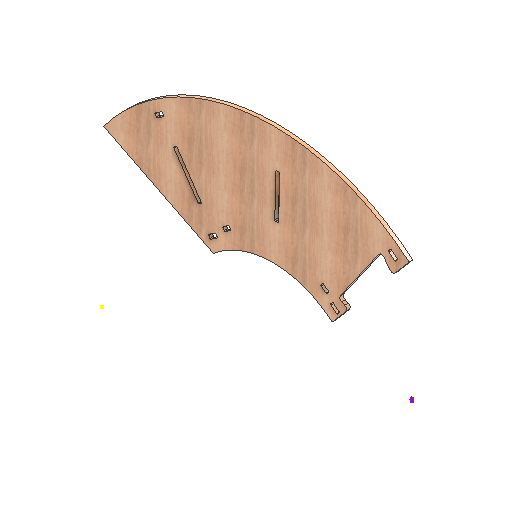
# Autodesk Inventor part: Platform B4
Saved by Autodesk Inventor 2021 (Build 250183000, 183)
## iProperties
Created: 2020-05-09
Part Number: Platform B4
Material: Wood (Birch)
Document SubType Name: Modeling
Designer: Dan Wikman
Density: 0.55 g/cm^3
Appearance: Birch - Natural Polished
Mass: 6310.79 g
Surface Area: 13696.6 cm^2
Volume: 11474.2 cm^3
Autodesk Inventor part; units mm, degrees
(part 1 of 2)
ref_plane "YZ Plane" through (0, 0, 0) normal (1, 0, 0) x (0, 1, 0)
ref_plane "XZ Plane" through (0, 0, 0) normal (0, 1, 0) x (-1, 0, 0)
ref_plane "XY Plane" through (0, 0, 0) normal (0, 0, 1) x (1, 0, 0)
sketch "Sketch1" plane through (0, 0, 0) normal (0, 0, 1) x (1, 0, 0)
  point P0 (0, 0)
sketch "CONTOURS" plane through (0, 0, 0) normal (0, 0, 1) x (1, 0, 0)
  line L0 (890.613, 255.6505) -> (890.613, 225.6505)
  line L1 (1985, 997.9541) -> (1985, 982.2281)
  arc A0 (1985, 982.2281) -> (1987, 980.2277) centre (1987, 982.2277) ccw
  line L2 (1987, 980.2277) -> (2103, 980.2277)
  arc A1 (2103, 980.2277) -> (2105, 982.2277) centre (2103, 982.2277) ccw
  line L3 (2105, 982.2277) -> (2105, 988.2874)
  arc A2 (2105, 988.2874) -> (2103.1661, 990.2805) centre (2103, 988.2874) ccw
  line L4 (2103.1661, 990.2805) -> (1987.1661, 999.9472)
  arc A3 (1987.1661, 999.9472) -> (1985, 997.9541) centre (1987, 997.9541) ccw
  line L5 (2105.3322, 1032.9996) -> (2105.3322, 1017.2736)
  arc A4 (2103.1661, 1015.2805) -> (2105.3322, 1017.2736) centre (2103.3322, 1017.2736) ccw
  line L6 (2103.1661, 1015.2805) -> (1987.1661, 1024.9472)
  arc A5 (1985.3322, 1026.9403) -> (1987.1661, 1024.9472) centre (1987.3322, 1026.9403) ccw
  line L7 (1985.3322, 1026.9403) -> (1985.3322, 1033)
  arc A6 (1987.3322, 1035) -> (1985.3322, 1033) centre (1987.3322, 1033) ccw
  line L8 (1987.3322, 1035) -> (2103.3322, 1035)
  arc A7 (2105.3322, 1032.9996) -> (2103.3322, 1035) centre (2103.3322, 1033) ccw
  line L9 (2125, 982.2281) -> (2125, 997.9541)
  arc A8 (2127.1661, 999.9472) -> (2125, 997.9541) centre (2127, 997.9541) ccw
  line L10 (2127.1661, 999.9472) -> (2243.1661, 990.2805)
  arc A9 (2245, 988.2874) -> (2243.1661, 990.2805) centre (2243, 988.2874) ccw
  line L11 (2245, 988.2874) -> (2245, 982.2277)
  arc A10 (2243, 980.2277) -> (2245, 982.2277) centre (2243, 982.2277) ccw
  line L12 (2243, 980.2277) -> (2127, 980.2277)
  arc A11 (2125, 982.2281) -> (2127, 980.2277) centre (2127, 982.2277) ccw
  line L13 (2265, 902.2281) -> (2265, 917.9541)
  arc A12 (2267.1661, 919.9472) -> (2265, 917.9541) centre (2267, 917.9541) ccw
  line L14 (2267.1661, 919.9472) -> (2383.1661, 910.2805)
  line L15 (2385, 908.2874) -> (2385, 902.2277)
  arc A13 (2383, 900.2277) -> (2385, 902.2277) centre (2383, 902.2277) ccw
  line L16 (2383, 900.2277) -> (2267, 900.2277)
  arc A14 (2265, 902.2281) -> (2267, 900.2277) centre (2267, 902.2277) ccw
  line L17 (2385.3322, 952.9996) -> (2385.3322, 937.2736)
  arc A15 (2383.1661, 935.2805) -> (2385.3322, 937.2736) centre (2383.3322, 937.2736) ccw
  line L18 (2383.1661, 935.2805) -> (2267.1661, 944.9472)
  arc A16 (2265.3322, 946.9403) -> (2267.1661, 944.9472) centre (2267.3322, 946.9403) ccw
  line L19 (2265.3322, 946.9403) -> (2265.3322, 953)
  arc A17 (2267.3322, 955) -> (2265.3322, 953) centre (2267.3322, 953) ccw
  line L20 (2267.3322, 955) -> (2383.3322, 955)
  arc A18 (2385.3322, 952.9996) -> (2383.3322, 955) centre (2383.3322, 953) ccw
  line L21 (2265, 1077.9541) -> (2265, 1062.2281)
  arc A19 (2265, 1062.2281) -> (2267, 1060.2277) centre (2267, 1062.2277) ccw
  line L22 (2267, 1060.2277) -> (2383, 1060.2277)
  arc A20 (2383, 1060.2277) -> (2385, 1062.2277) centre (2383, 1062.2277) ccw
  line L23 (2385, 1062.2277) -> (2385, 1068.2874)
  arc A21 (2385, 1068.2874) -> (2383.1661, 1070.2805) centre (2383, 1068.2874) ccw
  line L24 (2383.1661, 1070.2805) -> (2267.1661, 1079.9472)
  arc A22 (2267.1661, 1079.9472) -> (2265, 1077.9541) centre (2267, 1077.9541) ccw
  line L25 (2385.3322, 1112.9996) -> (2385.3322, 1097.2736)
  arc A23 (2383.1661, 1095.2805) -> (2385.3322, 1097.2736) centre (2383.3322, 1097.2736) ccw
  line L26 (2383.1661, 1095.2805) -> (2267.1661, 1104.9472)
  arc A24 (2265.3322, 1106.9403) -> (2267.1661, 1104.9472) centre (2267.3322, 1106.9403) ccw
  line L27 (2265.3322, 1106.9403) -> (2265.3322, 1113)
  arc A25 (2267.3322, 1115) -> (2265.3322, 1113) centre (2267.3322, 1113) ccw
  line L28 (2267.3322, 1115) -> (2383.3322, 1115)
  arc A26 (2385.3322, 1112.9996) -> (2383.3322, 1115) centre (2383.3322, 1113) ccw
  line L29 (2245.3322, 1112.9996) -> (2245.3322, 1097.2736)
  arc A27 (2243.1661, 1095.2805) -> (2245.3322, 1097.2736) centre (2243.3322, 1097.2736) ccw
  line L30 (2243.1661, 1095.2805) -> (2127.1661, 1104.9472)
  arc A28 (2125.3322, 1106.9403) -> (2127.1661, 1104.9472) centre (2127.3322, 1106.9403) ccw
  line L31 (2125.3322, 1106.9403) -> (2125.3322, 1113)
  arc A29 (2127.3322, 1115) -> (2125.3322, 1113) centre (2127.3322, 1113) ccw
  line L32 (2127.3322, 1115) -> (2243.3322, 1115)
  arc A30 (2245.3322, 1112.9996) -> (2243.3322, 1115) centre (2243.3322, 1113) ccw
  line L33 (2125, 1062.2281) -> (2125, 1077.9541)
  arc A31 (2127.1661, 1079.9472) -> (2125, 1077.9541) centre (2127, 1077.9541) ccw
  line L34 (2127.1661, 1079.9472) -> (2243.1661, 1070.2805)
  arc A32 (2245, 1068.2874) -> (2243.1661, 1070.2805) centre (2243, 1068.2874) ccw
  line L35 (2245, 1068.2874) -> (2245, 1062.2277)
  arc A33 (2243, 1060.2277) -> (2245, 1062.2277) centre (2243, 1062.2277) ccw
  line L36 (1397.2136, 921.0635) -> (1428.3528, 880.2176)
  arc A34 (1428.3528, 880.2176) -> (1450.9296, 879.6147) centre (1439.884, 889.0085) ccw
  line L37 (1450.9296, 879.6147) -> (1520.8494, 961.8291)
  arc A35 (1520.8494, 961.8291) -> (24.3664, 789.4308) centre (853.2136, 175.9412) ccw
  line L38 (24.3664, 789.4308) -> (562.1144, 519.2117)
  arc A36 (1144.4223, 519.2117) -> (562.1144, 519.2117) centre (853.2684, 176.0899) ccw
  line L39 (1144.4223, 519.2117) -> (1211.5255, 598.1141)
  arc A37 (1211.5255, 598.1141) -> (1206.0707, 620.8867) centre (1200.4798, 607.5079) ccw
  line L40 (1206.0707, 620.8867) -> (1190.5072, 627.3906)
  arc A38 (1183.7728, 650.5625) -> (1190.5072, 627.3906) centre (1196.4836, 641.6921) ccw
  line L41 (1183.7728, 650.5625) -> (1372.1762, 920.5366)
  arc A39 (1397.2136, 921.0635) -> (1372.1762, 920.5366) centre (1384.8871, 911.6663) ccw
  line L42 (2243, 1060.2277) -> (2127, 1060.2277)
  arc A40 (2125, 1062.2281) -> (2127, 1060.2277) centre (2127, 1062.2277) ccw
  line L43 (1985, 1077.9541) -> (1985, 1062.2281)
  arc A41 (1985, 1062.2281) -> (1987, 1060.2277) centre (1987, 1062.2277) ccw
  line L44 (1987, 1060.2277) -> (2103, 1060.2277)
  arc A42 (2103, 1060.2277) -> (2105, 1062.2277) centre (2103, 1062.2277) ccw
  line L45 (2105, 1062.2277) -> (2105, 1068.2874)
  arc A43 (2105, 1068.2874) -> (2103.1661, 1070.2805) centre (2103, 1068.2874) ccw
  line L46 (2103.1661, 1070.2805) -> (1987.1661, 1079.9472)
  arc A44 (1987.1661, 1079.9472) -> (1985, 1077.9541) centre (1987, 1077.9541) ccw
  line L47 (2385.3322, 1032.9996) -> (2385.3322, 1017.2736)
  arc A45 (2383.1661, 1015.2805) -> (2385.3322, 1017.2736) centre (2383.3322, 1017.2736) ccw
  line L48 (2383.1661, 1015.2805) -> (2267.1661, 1024.9472)
  arc A46 (2265.3322, 1026.9403) -> (2267.1661, 1024.9472) centre (2267.3322, 1026.9403) ccw
  line L49 (2265.3322, 1026.9403) -> (2265.3322, 1033)
  arc A47 (2267.3322, 1035) -> (2265.3322, 1033) centre (2267.3322, 1033) ccw
  line L50 (2267.3322, 1035) -> (2383.3322, 1035)
  arc A48 (2385.3322, 1032.9996) -> (2383.3322, 1035) centre (2383.3322, 1033) ccw
  line L51 (2245.3322, 1032.9996) -> (2245.3322, 1017.2736)
  arc A49 (2243.1661, 1015.2805) -> (2245.3322, 1017.2736) centre (2243.3322, 1017.2736) ccw
  line L52 (2243.1661, 1015.2805) -> (2127.1661, 1024.9472)
  arc A50 (1985.3322, 866.9403) -> (1987.1661, 864.9472) centre (1987.3322, 866.9403) ccw
  arc A51 (2125.3322, 1026.9403) -> (2127.1661, 1024.9472) centre (2127.3322, 1026.9403) ccw
  line L53 (2125.3322, 1026.9403) -> (2125.3322, 1033)
  line L54 (2153.8888, 619.2359) -> (2163.4719, 633.117)
  arc A52 (2185.9832, 634.7957) -> (2163.4719, 633.117) centre (2175.4045, 624.8791) ccw
  line L55 (2185.9832, 634.7957) -> (2411.1355, 394.6117)
  arc A53 (2406.7717, 371.5944) -> (2411.1355, 394.6117) centre (2400.5567, 384.695) ccw
  line L56 (2406.7717, 371.5944) -> (2360.367, 349.5799)
  arc A54 (2360.367, 349.5799) -> (2354.7432, 326.1016) centre (2367.0105, 335.5759) ccw
  line L57 (2354.7432, 326.1016) -> (2420.766, 240.6152)
  arc A55 (991.9076, 405.3519) -> (2420.766, 240.6152) centre (1790.9625, 1056.9921) ccw
  line L58 (991.9076, 405.3519) -> (1516.221, 700.5434)
  arc A56 (1516.221, 700.5434) -> (2065.5544, 700.5434) centre (1790.8877, 1057.1243) ccw
  line L59 (2065.5544, 700.5434) -> (2128.8659, 618.5677)
  arc A57 (2128.8659, 618.5677) -> (2153.8888, 619.2359) centre (2141.1332, 628.042) ccw
  arc A58 (2127.3322, 1035) -> (2125.3322, 1033) centre (2127.3322, 1033) ccw
  line L60 (2127.3322, 1035) -> (2243.3322, 1035)
  arc A59 (2245.3322, 1032.9996) -> (2243.3322, 1035) centre (2243.3322, 1033) ccw
  line L61 (2105.3322, 1112.9996) -> (2105.3322, 1097.2736)
  arc A60 (2103.1661, 1095.2805) -> (2105.3322, 1097.2736) centre (2103.3322, 1097.2736) ccw
  line L62 (2103.1661, 1095.2805) -> (1987.1661, 1104.9472)
  arc A61 (1985.3322, 1106.9403) -> (1987.1661, 1104.9472) centre (1987.3322, 1106.9403) ccw
  line L63 (1985.3322, 1106.9403) -> (1985.3322, 1113)
  arc A62 (1987.3322, 1115) -> (1985.3322, 1113) centre (1987.3322, 1113) ccw
  line L64 (1987.3322, 1115) -> (2103.3322, 1115)
  arc A63 (2105.3322, 1112.9996) -> (2103.3322, 1115) centre (2103.3322, 1113) ccw
  line L65 (2245.3322, 952.9996) -> (2245.3322, 937.2736)
  arc A64 (2243.1661, 935.2805) -> (2245.3322, 937.2736) centre (2243.3322, 937.2736) ccw
  line L66 (2243.1661, 935.2805) -> (2127.1661, 944.9472)
  arc A65 (2125.3322, 946.9403) -> (2127.1661, 944.9472) centre (2127.3322, 946.9403) ccw
  line L67 (2125.3322, 946.9403) -> (2125.3322, 953)
  arc A66 (2127.3322, 955) -> (2125.3322, 953) centre (2127.3322, 953) ccw
  line L68 (2127.3322, 955) -> (2243.3322, 955)
  arc A67 (2245.3322, 952.9996) -> (2243.3322, 955) centre (2243.3322, 953) ccw
  arc A68 (2385, 908.2874) -> (2383.1661, 910.2805) centre (2383, 908.2874) ccw
  arc A69 (113.8436, 518.7397) -> (113.8436, 526.7397) centre (113.8436, 522.7397) ccw
  line L69 (113.8436, 526.7397) -> (113.8436, 528.7397)
  line L70 (113.8436, 528.7397) -> (472.3436, 528.7397)
  line L71 (472.3436, 528.7397) -> (472.3436, 526.7397)
  arc A70 (472.3436, 526.7397) -> (472.3436, 518.7397) centre (472.3436, 522.7397) ccw
  line L72 (472.3436, 518.7397) -> (490.3436, 518.7397)
  line L73 (490.3436, 518.7397) -> (490.3436, 488.7397)
  line L74 (490.3436, 488.7397) -> (472.3436, 488.7397)
  arc A71 (472.3436, 488.7397) -> (472.3436, 480.7397) centre (472.3436, 484.7397) ccw
  line L75 (472.3436, 480.7397) -> (472.3436, 428.7397)
  line L76 (472.3436, 428.7397) -> (301.0936, 428.7397)
  arc A72 (301.0936, 428.7397) -> (293.0936, 428.7397) centre (297.0936, 428.7397) ccw
  line L77 (293.0936, 428.7397) -> (293.0936, 410.7397)
  line L78 (293.0936, 410.7397) -> (263.0936, 410.7397)
  line L79 (263.0936, 410.7397) -> (263.0936, 428.7397)
  arc A73 (263.0936, 428.7397) -> (255.0936, 428.7397) centre (259.0936, 428.7397) ccw
  line L80 (255.0936, 428.7397) -> (113.8436, 428.7397)
  line L81 (113.8436, 428.7397) -> (113.8436, 480.7397)
  arc A74 (113.8436, 480.7397) -> (113.8436, 488.7397) centre (113.8436, 484.7397) ccw
  line L82 (113.8436, 488.7397) -> (95.8436, 488.7397)
  line L83 (95.8436, 488.7397) -> (95.8436, 518.7397)
  line L84 (95.8436, 518.7397) -> (113.8436, 518.7397)
  arc A75 (87.6316, 255.6505) -> (87.6316, 263.6505) centre (87.6316, 259.6505) ccw
  line L85 (87.6316, 263.6505) -> (87.6316, 265.6505)
  line L86 (87.6316, 265.6505) -> (446.1316, 265.6505)
  line L87 (446.1316, 265.6505) -> (446.1316, 263.6505)
  arc A76 (446.1316, 263.6505) -> (446.1316, 255.6505) centre (446.1316, 259.6505) ccw
  line L88 (446.1316, 255.6505) -> (464.1316, 255.6505)
  line L89 (464.1316, 255.6505) -> (464.1316, 225.6505)
  line L90 (464.1316, 225.6505) -> (446.1316, 225.6505)
  arc A77 (446.1316, 225.6505) -> (446.1316, 217.6505) centre (446.1316, 221.6505) ccw
  line L91 (446.1316, 217.6505) -> (446.1316, 165.6505)
  line L92 (446.1316, 165.6505) -> (274.8816, 165.6505)
  arc A78 (274.8816, 165.6505) -> (266.8816, 165.6505) centre (270.8816, 165.6505) ccw
  line L93 (266.8816, 165.6505) -> (266.8816, 147.6505)
  line L94 (266.8816, 147.6505) -> (236.8816, 147.6505)
  line L95 (236.8816, 147.6505) -> (236.8816, 165.6505)
  arc A79 (236.8816, 165.6505) -> (228.8816, 165.6505) centre (232.8816, 165.6505) ccw
  line L96 (228.8816, 165.6505) -> (87.6316, 165.6505)
  line L97 (87.6316, 165.6505) -> (87.6316, 217.6505)
  arc A80 (87.6316, 217.6505) -> (87.6316, 225.6505) centre (87.6316, 221.6505) ccw
  line L98 (87.6316, 225.6505) -> (69.6316, 225.6505)
  line L99 (69.6316, 225.6505) -> (69.6316, 255.6505)
  line L100 (69.6316, 255.6505) -> (87.6316, 255.6505)
  arc A81 (514.113, 255.6505) -> (514.113, 263.6505) centre (514.113, 259.6505) ccw
  line L101 (514.113, 263.6505) -> (514.113, 265.6505)
  line L102 (514.113, 265.6505) -> (872.613, 265.6505)
  line L103 (872.613, 265.6505) -> (872.613, 263.6505)
  arc A82 (872.613, 263.6505) -> (872.613, 255.6505) centre (872.613, 259.6505) ccw
  line L104 (872.613, 255.6505) -> (890.613, 255.6505)
  line L105 (890.613, 225.6505) -> (872.613, 225.6505)
  arc A83 (872.613, 225.6505) -> (872.613, 217.6505) centre (872.613, 221.6505) ccw
  line L106 (872.613, 217.6505) -> (872.613, 165.6505)
  line L107 (872.613, 165.6505) -> (701.363, 165.6505)
  arc A84 (701.363, 165.6505) -> (693.363, 165.6505) centre (697.363, 165.6505) ccw
  line L108 (693.363, 165.6505) -> (693.363, 147.6505)
  line L109 (693.363, 147.6505) -> (663.363, 147.6505)
  line L110 (663.363, 147.6505) -> (663.363, 165.6505)
  arc A85 (663.363, 165.6505) -> (655.363, 165.6505) centre (659.363, 165.6505) ccw
  line L111 (655.363, 165.6505) -> (514.113, 165.6505)
  line L112 (514.113, 165.6505) -> (514.113, 217.6505)
  arc A86 (514.113, 217.6505) -> (514.113, 225.6505) centre (514.113, 221.6505) ccw
  line L113 (514.113, 225.6505) -> (496.113, 225.6505)
  line L114 (496.113, 225.6505) -> (496.113, 255.6505)
  line L115 (496.113, 255.6505) -> (514.113, 255.6505)
  arc A87 (616.5794, 518.7397) -> (616.5794, 526.7397) centre (616.5794, 522.7397) ccw
  line L116 (616.5794, 526.7397) -> (616.5794, 528.7397)
  line L117 (616.5794, 528.7397) -> (975.0794, 528.7397)
  line L118 (975.0794, 528.7397) -> (975.0794, 526.7397)
  arc A88 (975.0794, 526.7397) -> (975.0794, 518.7397) centre (975.0794, 522.7397) ccw
  line L119 (975.0794, 518.7397) -> (993.0794, 518.7397)
  line L120 (993.0794, 518.7397) -> (993.0794, 488.7397)
  line L121 (993.0794, 488.7397) -> (975.0794, 488.7397)
  arc A89 (975.0794, 488.7397) -> (975.0794, 480.7397) centre (975.0794, 484.7397) ccw
  line L122 (975.0794, 480.7397) -> (975.0794, 428.7397)
  line L123 (975.0794, 428.7397) -> (803.8294, 428.7397)
  arc A90 (803.8294, 428.7397) -> (795.8294, 428.7397) centre (799.8294, 428.7397) ccw
  line L124 (795.8294, 428.7397) -> (795.8294, 410.7397)
  line L125 (795.8294, 410.7397) -> (765.8294, 410.7397)
  line L126 (765.8294, 410.7397) -> (765.8294, 428.7397)
  arc A91 (765.8294, 428.7397) -> (757.8294, 428.7397) centre (761.8294, 428.7397) ccw
  line L127 (757.8294, 428.7397) -> (616.5794, 428.7397)
  line L128 (616.5794, 428.7397) -> (616.5794, 480.7397)
  arc A92 (616.5794, 480.7397) -> (616.5794, 488.7397) centre (616.5794, 484.7397) ccw
  line L129 (616.5794, 488.7397) -> (598.5794, 488.7397)
  line L130 (598.5794, 488.7397) -> (598.5794, 518.7397)
  line L131 (598.5794, 518.7397) -> (616.5794, 518.7397)
  arc A93 (464.113, 29.6505) -> (464.113, 37.6505) centre (464.113, 33.6505) ccw
  line L132 (464.113, 29.6505) -> (464.113, 27.6505)
  line L133 (464.113, 27.6505) -> (822.613, 27.6505)
  line L134 (822.613, 27.6505) -> (822.613, 29.6505)
  arc A94 (822.613, 37.6505) -> (822.613, 29.6505) centre (822.613, 33.6505) ccw
  line L135 (822.613, 37.6505) -> (840.613, 37.6505)
  line L136 (840.613, 37.6505) -> (840.613, 67.6505)
  line L137 (840.613, 67.6505) -> (822.613, 67.6505)
  arc A95 (822.613, 75.6505) -> (822.613, 67.6505) centre (822.613, 71.6505) ccw
  line L138 (822.613, 75.6505) -> (822.613, 127.6505)
  line L139 (822.613, 127.6505) -> (651.363, 127.6505)
  arc A96 (643.363, 127.6505) -> (651.363, 127.6505) centre (647.363, 127.6505) ccw
  line L140 (643.363, 127.6505) -> (643.363, 145.6505)
  line L141 (643.363, 145.6505) -> (613.363, 145.6505)
  line L142 (613.363, 145.6505) -> (613.363, 127.6505)
  arc A97 (605.363, 127.6505) -> (613.363, 127.6505) centre (609.363, 127.6505) ccw
  line L143 (605.363, 127.6505) -> (464.113, 127.6505)
  line L144 (464.113, 127.6505) -> (464.113, 75.6505)
  arc A98 (464.113, 67.6505) -> (464.113, 75.6505) centre (464.113, 71.6505) ccw
  line L145 (464.113, 67.6505) -> (446.113, 67.6505)
  line L146 (446.113, 67.6505) -> (446.113, 37.6505)
  line L147 (446.113, 37.6505) -> (464.113, 37.6505)
  arc A99 (37.6316, 29.6505) -> (37.6316, 37.6505) centre (37.6316, 33.6505) ccw
  line L148 (37.6316, 29.6505) -> (37.6316, 27.6505)
  line L149 (37.6316, 27.6505) -> (396.1316, 27.6505)
  line L150 (396.1316, 27.6505) -> (396.1316, 29.6505)
  arc A100 (396.1316, 37.6505) -> (396.1316, 29.6505) centre (396.1316, 33.6505) ccw
  line L151 (396.1316, 37.6505) -> (414.1316, 37.6505)
  line L152 (414.1316, 37.6505) -> (414.1316, 67.6505)
  line L153 (414.1316, 67.6505) -> (396.1316, 67.6505)
  arc A101 (396.1316, 75.6505) -> (396.1316, 67.6505) centre (396.1316, 71.6505) ccw
  line L154 (396.1316, 75.6505) -> (396.1316, 127.6505)
  line L155 (396.1316, 127.6505) -> (224.8816, 127.6505)
  arc A102 (216.8816, 127.6505) -> (224.8816, 127.6505) centre (220.8816, 127.6505) ccw
  line L156 (216.8816, 127.6505) -> (216.8816, 145.6505)
  line L157 (216.8816, 145.6505) -> (186.8816, 145.6505)
  line L158 (186.8816, 145.6505) -> (186.8816, 127.6505)
  arc A103 (178.8816, 127.6505) -> (186.8816, 127.6505) centre (182.8816, 127.6505) ccw
  line L159 (178.8816, 127.6505) -> (37.6316, 127.6505)
  line L160 (37.6316, 127.6505) -> (37.6316, 75.6505)
  arc A104 (37.6316, 67.6505) -> (37.6316, 75.6505) centre (37.6316, 71.6505) ccw
  line L161 (37.6316, 67.6505) -> (19.6316, 67.6505)
  line L162 (19.6316, 67.6505) -> (19.6316, 37.6505)
  line L163 (19.6316, 37.6505) -> (37.6316, 37.6505)
  arc A105 (566.5794, 292.7397) -> (566.5794, 300.7397) centre (566.5794, 296.7397) ccw
  line L164 (566.5794, 292.7397) -> (566.5794, 290.7397)
  line L165 (566.5794, 290.7397) -> (925.0794, 290.7397)
  line L166 (925.0794, 290.7397) -> (925.0794, 292.7397)
  arc A106 (925.0794, 300.7397) -> (925.0794, 292.7397) centre (925.0794, 296.7397) ccw
  line L167 (925.0794, 300.7397) -> (943.0794, 300.7397)
  line L168 (943.0794, 300.7397) -> (943.0794, 330.7397)
  line L169 (943.0794, 330.7397) -> (925.0794, 330.7397)
  arc A107 (925.0794, 338.7397) -> (925.0794, 330.7397) centre (925.0794, 334.7397) ccw
  line L170 (925.0794, 338.7397) -> (925.0794, 390.7397)
  line L171 (925.0794, 390.7397) -> (753.8294, 390.7397)
  arc A108 (745.8294, 390.7397) -> (753.8294, 390.7397) centre (749.8294, 390.7397) ccw
  line L172 (745.8294, 390.7397) -> (745.8294, 408.7397)
  line L173 (745.8294, 408.7397) -> (715.8294, 408.7397)
  line L174 (715.8294, 408.7397) -> (715.8294, 390.7397)
  arc A109 (707.8294, 390.7397) -> (715.8294, 390.7397) centre (711.8294, 390.7397) ccw
  line L175 (707.8294, 390.7397) -> (566.5794, 390.7397)
  line L176 (566.5794, 390.7397) -> (566.5794, 338.7397)
  arc A110 (566.5794, 330.7397) -> (566.5794, 338.7397) centre (566.5794, 334.7397) ccw
  line L177 (566.5794, 330.7397) -> (548.5794, 330.7397)
  line L178 (548.5794, 330.7397) -> (548.5794, 300.7397)
  line L179 (548.5794, 300.7397) -> (566.5794, 300.7397)
  arc A111 (63.8436, 292.7397) -> (63.8436, 300.7397) centre (63.8436, 296.7397) ccw
  line L180 (63.8436, 292.7397) -> (63.8436, 290.7397)
  line L181 (63.8436, 290.7397) -> (422.3436, 290.7397)
  line L182 (422.3436, 290.7397) -> (422.3436, 292.7397)
  arc A112 (422.3436, 300.7397) -> (422.3436, 292.7397) centre (422.3436, 296.7397) ccw
  line L183 (422.3436, 300.7397) -> (440.3436, 300.7397)
  line L184 (440.3436, 300.7397) -> (440.3436, 330.7397)
  line L185 (440.3436, 330.7397) -> (422.3436, 330.7397)
  arc A113 (422.3436, 338.7397) -> (422.3436, 330.7397) centre (422.3436, 334.7397) ccw
  line L186 (422.3436, 338.7397) -> (422.3436, 390.7397)
  line L187 (422.3436, 390.7397) -> (251.0936, 390.7397)
  arc A114 (243.0936, 390.7397) -> (251.0936, 390.7397) centre (247.0936, 390.7397) ccw
  line L188 (243.0936, 390.7397) -> (243.0936, 408.7397)
  line L189 (243.0936, 408.7397) -> (213.0936, 408.7397)
  line L190 (213.0936, 408.7397) -> (213.0936, 390.7397)
  arc A115 (205.0936, 390.7397) -> (213.0936, 390.7397) centre (209.0936, 390.7397) ccw
  line L191 (205.0936, 390.7397) -> (63.8436, 390.7397)
  line L192 (63.8436, 390.7397) -> (63.8436, 338.7397)
  arc A116 (63.8436, 330.7397) -> (63.8436, 338.7397) centre (63.8436, 334.7397) ccw
  line L193 (63.8436, 330.7397) -> (45.8436, 330.7397)
  line L194 (45.8436, 330.7397) -> (45.8436, 300.7397)
  line L195 (45.8436, 300.7397) -> (63.8436, 300.7397)
  line L196 (1685.3322, 952.9996) -> (1685.3322, 937.2736)
  arc A117 (1683.1661, 935.2805) -> (1685.3322, 937.2736) centre (1683.3322, 937.2736) ccw
  line L197 (1683.1661, 935.2805) -> (1567.1661, 944.9472)
  arc A118 (1565.3322, 946.9403) -> (1567.1661, 944.9472) centre (1567.3322, 946.9403) ccw
  line L198 (1565.3322, 946.9403) -> (1565.3322, 953)
  arc A119 (1567.3322, 955) -> (1565.3322, 953) centre (1567.3322, 953) ccw
  line L199 (1567.3322, 955) -> (1683.3322, 955)
  arc A120 (1685.3322, 952.9996) -> (1683.3322, 955) centre (1683.3322, 953) ccw
  line L200 (1565, 902.2281) -> (1565, 917.9541)
  arc A121 (1567.1661, 919.9472) -> (1565, 917.9541) centre (1567, 917.9541) ccw
  line L201 (1567.1661, 919.9472) -> (1683.1661, 910.2805)
  arc A122 (1685, 908.2874) -> (1683.1661, 910.2805) centre (1683, 908.2874) ccw
  line L202 (1685, 908.2874) -> (1685, 902.2277)
  arc A123 (1683, 900.2277) -> (1685, 902.2277) centre (1683, 902.2277) ccw
  line L203 (1683, 900.2277) -> (1567, 900.2277)
  arc A124 (1565, 902.2281) -> (1567, 900.2277) centre (1567, 902.2277) ccw
  line L204 (2385.3322, 792.9996) -> (2385.3322, 777.2736)
  arc A125 (2383.1661, 775.2805) -> (2385.3322, 777.2736) centre (2383.3322, 777.2736) ccw
  line L205 (2383.1661, 775.2805) -> (2267.1661, 784.9472)
  arc A126 (2265.3322, 786.9403) -> (2267.1661, 784.9472) centre (2267.3322, 786.9403) ccw
  line L206 (2265.3322, 786.9403) -> (2265.3322, 793)
  arc A127 (2267.3322, 795) -> (2265.3322, 793) centre (2267.3322, 793) ccw
  line L207 (2267.3322, 795) -> (2383.3322, 795)
  arc A128 (2385.3322, 792.9996) -> (2383.3322, 795) centre (2383.3322, 793) ccw
  line L208 (2265, 742.2281) -> (2265, 757.9541)
  arc A129 (2267.1661, 759.9472) -> (2265, 757.9541) centre (2267, 757.9541) ccw
  line L209 (2267.1661, 759.9472) -> (2383.1661, 750.2805)
  arc A130 (2385, 748.2874) -> (2383.1661, 750.2805) centre (2383, 748.2874) ccw
  line L210 (2385, 748.2874) -> (2385, 742.2277)
  arc A131 (2383, 740.2277) -> (2385, 742.2277) centre (2383, 742.2277) ccw
  line L211 (2383, 740.2277) -> (2267, 740.2277)
  arc A132 (2265, 742.2281) -> (2267, 740.2277) centre (2267, 742.2277) ccw
  line L212 (1705, 982.2281) -> (1705, 997.9541)
  arc A133 (1707.1661, 999.9472) -> (1705, 997.9541) centre (1707, 997.9541) ccw
  line L213 (1707.1661, 999.9472) -> (1823.1661, 990.2805)
  arc A134 (1825, 988.2874) -> (1823.1661, 990.2805) centre (1823, 988.2874) ccw
  line L214 (1825, 988.2874) -> (1825, 982.2277)
  arc A135 (1823, 980.2277) -> (1825, 982.2277) centre (1823, 982.2277) ccw
  line L215 (1823, 980.2277) -> (1707, 980.2277)
  arc A136 (1705, 982.2281) -> (1707, 980.2277) centre (1707, 982.2277) ccw
  line L216 (1685.3322, 1032.9996) -> (1685.3322, 1017.2736)
  arc A137 (1683.1661, 1015.2805) -> (1685.3322, 1017.2736) centre (1683.3322, 1017.2736) ccw
  line L217 (1683.1661, 1015.2805) -> (1567.1661, 1024.9472)
  arc A138 (1565.3322, 1026.9403) -> (1567.1661, 1024.9472) centre (1567.3322, 1026.9403) ccw
  line L218 (1565.3322, 1026.9403) -> (1565.3322, 1033)
  arc A139 (1567.3322, 1035) -> (1565.3322, 1033) centre (1567.3322, 1033) ccw
  line L219 (1567.3322, 1035) -> (1683.3322, 1035)
  arc A140 (1685.3322, 1032.9996) -> (1683.3322, 1035) centre (1683.3322, 1033) ccw
  line L220 (2385.3322, 872.9996) -> (2385.3322, 857.2736)
  arc A141 (2383.1661, 855.2805) -> (2385.3322, 857.2736) centre (2383.3322, 857.2736) ccw
  line L221 (2383.1661, 855.2805) -> (2267.1661, 864.9472)
  arc A142 (2265.3322, 866.9403) -> (2267.1661, 864.9472) centre (2267.3322, 866.9403) ccw
  line L222 (2265.3322, 866.9403) -> (2265.3322, 873)
  arc A143 (2267.3322, 875) -> (2265.3322, 873) centre (2267.3322, 873) ccw
  line L223 (2267.3322, 875) -> (2383.3322, 875)
  arc A144 (2385.3322, 872.9996) -> (2383.3322, 875) centre (2383.3322, 873) ccw
  line L224 (1565, 997.9541) -> (1565, 982.2281)
  arc A145 (1565, 982.2281) -> (1567, 980.2277) centre (1567, 982.2277) ccw
  line L225 (1567, 980.2277) -> (1683, 980.2277)
  arc A146 (1683, 980.2277) -> (1685, 982.2277) centre (1683, 982.2277) ccw
  line L226 (1685, 982.2277) -> (1685, 988.2874)
  arc A147 (1685, 988.2874) -> (1683.1661, 990.2805) centre (1683, 988.2874) ccw
  line L227 (1683.1661, 990.2805) -> (1567.1661, 999.9472)
  arc A148 (1567.1661, 999.9472) -> (1565, 997.9541) centre (1567, 997.9541) ccw
  line L228 (2265, 822.2281) -> (2265, 837.9541)
  arc A149 (2267.1661, 839.9472) -> (2265, 837.9541) centre (2267, 837.9541) ccw
  line L229 (2267.1661, 839.9472) -> (2383.1661, 830.2805)
  arc A150 (2385, 828.2874) -> (2383.1661, 830.2805) centre (2383, 828.2874) ccw
  line L230 (2385, 828.2874) -> (2385, 822.2277)
  arc A151 (2383, 820.2277) -> (2385, 822.2277) centre (2383, 822.2277) ccw
  line L231 (2383, 820.2277) -> (2267, 820.2277)
  arc A152 (2265, 822.2281) -> (2267, 820.2277) centre (2267, 822.2277) ccw
  line L232 (1965.3322, 792.9996) -> (1965.3322, 777.2736)
  arc A153 (1963.1661, 775.2805) -> (1965.3322, 777.2736) centre (1963.3322, 777.2736) ccw
  line L233 (1963.1661, 775.2805) -> (1847.1661, 784.9472)
  arc A154 (1845.3322, 786.9403) -> (1847.1661, 784.9472) centre (1847.3322, 786.9403) ccw
  line L234 (1845.3322, 786.9403) -> (1845.3322, 793)
  arc A155 (1847.3322, 795) -> (1845.3322, 793) centre (1847.3322, 793) ccw
  line L235 (1847.3322, 795) -> (1963.3322, 795)
  arc A156 (1965.3322, 792.9996) -> (1963.3322, 795) centre (1963.3322, 793) ccw
  line L236 (2105.3322, 872.9996) -> (2105.3322, 857.2736)
  arc A157 (2103.1661, 855.2805) -> (2105.3322, 857.2736) centre (2103.3322, 857.2736) ccw
  line L237 (2103.1661, 855.2805) -> (1987.1661, 864.9472)
  line L238 (2105, 748.2874) -> (2105, 742.2277)
  line L239 (1985.3322, 866.9403) -> (1985.3322, 873)
  arc A158 (1987.3322, 875) -> (1985.3322, 873) centre (1987.3322, 873) ccw
  line L240 (1987.3322, 875) -> (2103.3322, 875)
  arc A159 (2105.3322, 872.9996) -> (2103.3322, 875) centre (2103.3322, 873) ccw
  line L241 (1565, 1077.9541) -> (1565, 1062.2281)
  arc A160 (1565, 1062.2281) -> (1567, 1060.2277) centre (1567, 1062.2277) ccw
  line L242 (1567, 1060.2277) -> (1683, 1060.2277)
  arc A161 (1683, 1060.2277) -> (1685, 1062.2277) centre (1683, 1062.2277) ccw
  line L243 (1685, 1062.2277) -> (1685, 1068.2874)
  arc A162 (1685, 1068.2874) -> (1683.1661, 1070.2805) centre (1683, 1068.2874) ccw
  line L244 (1683.1661, 1070.2805) -> (1567.1661, 1079.9472)
  arc A163 (1567.1661, 1079.9472) -> (1565, 1077.9541) centre (1567, 1077.9541) ccw
  line L245 (1685.3322, 1112.9996) -> (1685.3322, 1097.2736)
  arc A164 (1683.1661, 1095.2805) -> (1685.3322, 1097.2736) centre (1683.3322, 1097.2736) ccw
  line L246 (1683.1661, 1095.2805) -> (1567.1661, 1104.9472)
  arc A165 (1565.3322, 1106.9403) -> (1567.1661, 1104.9472) centre (1567.3322, 1106.9403) ccw
  line L247 (1565.3322, 1106.9403) -> (1565.3322, 1113)
  arc A166 (1567.3322, 1115) -> (1565.3322, 1113) centre (1567.3322, 1113) ccw
  line L248 (1567.3322, 1115) -> (1683.3322, 1115)
  arc A167 (1685.3322, 1112.9996) -> (1683.3322, 1115) centre (1683.3322, 1113) ccw
  line L249 (1985, 837.9541) -> (1985, 822.2281)
  arc A168 (1985, 822.2281) -> (1987, 820.2277) centre (1987, 822.2277) ccw
  line L250 (1987, 820.2277) -> (2103, 820.2277)
  arc A169 (2103, 820.2277) -> (2105, 822.2277) centre (2103, 822.2277) ccw
  line L251 (2105, 822.2277) -> (2105, 828.2874)
  arc A170 (2105, 828.2874) -> (2103.1661, 830.2805) centre (2103, 828.2874) ccw
  line L252 (2103.1661, 830.2805) -> (1987.1661, 839.9472)
  arc A171 (1987.1661, 839.9472) -> (1985, 837.9541) centre (1987, 837.9541) ccw
  line L253 (1965.3322, 872.9996) -> (1965.3322, 857.2736)
  arc A172 (1963.1661, 855.2805) -> (1965.3322, 857.2736) centre (1963.3322, 857.2736) ccw
  line L254 (1963.1661, 855.2805) -> (1847.1661, 864.9472)
  arc A173 (1845.3322, 866.9403) -> (1847.1661, 864.9472) centre (1847.3322, 866.9403) ccw
  line L255 (1845.3322, 866.9403) -> (1845.3322, 873)
  arc A174 (1847.3322, 875) -> (1845.3322, 873) centre (1847.3322, 873) ccw
  line L256 (1847.3322, 875) -> (1963.3322, 875)
  arc A175 (1965.3322, 872.9996) -> (1963.3322, 875) centre (1963.3322, 873) ccw
  line L257 (1705, 902.2281) -> (1705, 917.9541)
  arc A176 (1707.1661, 919.9472) -> (1705, 917.9541) centre (1707, 917.9541) ccw
  line L258 (1707.1661, 919.9472) -> (1823.1661, 910.2805)
  arc A177 (1825, 908.2874) -> (1823.1661, 910.2805) centre (1823, 908.2874) ccw
  line L259 (1825, 908.2874) -> (1825, 902.2277)
  arc A178 (1823, 900.2277) -> (1825, 902.2277) centre (1823, 902.2277) ccw
  line L260 (1823, 900.2277) -> (1707, 900.2277)
  arc A179 (1705, 902.2281) -> (1707, 900.2277) centre (1707, 902.2277) ccw
  line L261 (1825.3322, 952.9996) -> (1825.3322, 937.2736)
  arc A180 (1823.1661, 935.2805) -> (1825.3322, 937.2736) centre (1823.3322, 937.2736) ccw
  line L262 (1823.1661, 935.2805) -> (1707.1661, 944.9472)
  arc A181 (1705.3322, 946.9403) -> (1707.1661, 944.9472) centre (1707.3322, 946.9403) ccw
  line L263 (1705.3322, 946.9403) -> (1705.3322, 953)
  arc A182 (1707.3322, 955) -> (1705.3322, 953) centre (1707.3322, 953) ccw
  line L264 (1707.3322, 955) -> (1823.3322, 955)
  arc A183 (1825.3322, 952.9996) -> (1823.3322, 955) centre (1823.3322, 953) ccw
  line L265 (1685.3322, 792.9996) -> (1685.3322, 777.2736)
  arc A184 (1683.1661, 775.2805) -> (1685.3322, 777.2736) centre (1683.3322, 777.2736) ccw
  line L266 (1683.1661, 775.2805) -> (1567.1661, 784.9472)
  arc A185 (1565.3322, 786.9403) -> (1567.1661, 784.9472) centre (1567.3322, 786.9403) ccw
  line L267 (1565.3322, 786.9403) -> (1565.3322, 793)
  arc A186 (1567.3322, 795) -> (1565.3322, 793) centre (1567.3322, 793) ccw
  line L268 (1567.3322, 795) -> (1683.3322, 795)
  arc A187 (1685.3322, 792.9996) -> (1683.3322, 795) centre (1683.3322, 793) ccw
  line L269 (1825.3322, 1032.9996) -> (1825.3322, 1017.2736)
  arc A188 (1823.1661, 1015.2805) -> (1825.3322, 1017.2736) centre (1823.3322, 1017.2736) ccw
  line L270 (1823.1661, 1015.2805) -> (1707.1661, 1024.9472)
  arc A189 (1705.3322, 1026.9403) -> (1707.1661, 1024.9472) centre (1707.3322, 1026.9403) ccw
  line L271 (1705.3322, 1026.9403) -> (1705.3322, 1033)
  arc A190 (1707.3322, 1035) -> (1705.3322, 1033) centre (1707.3322, 1033) ccw
  line L272 (1707.3322, 1035) -> (1823.3322, 1035)
  arc A191 (1825.3322, 1032.9996) -> (1823.3322, 1035) centre (1823.3322, 1033) ccw
  line L273 (1685.3322, 872.9996) -> (1685.3322, 857.2736)
  arc A192 (1683.1661, 855.2805) -> (1685.3322, 857.2736) centre (1683.3322, 857.2736) ccw
  line L274 (1683.1661, 855.2805) -> (1567.1661, 864.9472)
  arc A193 (1565.3322, 866.9403) -> (1567.1661, 864.9472) centre (1567.3322, 866.9403) ccw
  line L275 (1565.3322, 866.9403) -> (1565.3322, 873)
  arc A194 (1567.3322, 875) -> (1565.3322, 873) centre (1567.3322, 873) ccw
  line L276 (1567.3322, 875) -> (1683.3322, 875)
  arc A195 (1685.3322, 872.9996) -> (1683.3322, 875) centre (1683.3322, 873) ccw
  line L277 (1705, 1062.2281) -> (1705, 1077.9541)
  arc A196 (1707.1661, 1079.9472) -> (1705, 1077.9541) centre (1707, 1077.9541) ccw
  line L278 (1707.1661, 1079.9472) -> (1823.1661, 1070.2805)
  arc A197 (1825, 1068.2874) -> (1823.1661, 1070.2805) centre (1823, 1068.2874) ccw
  line L279 (1825, 1068.2874) -> (1825, 1062.2277)
  arc A198 (1823, 1060.2277) -> (1825, 1062.2277) centre (1823, 1062.2277) ccw
  line L280 (1823, 1060.2277) -> (1707, 1060.2277)
  arc A199 (1705, 1062.2281) -> (1707, 1060.2277) centre (1707, 1062.2277) ccw
  line L281 (1565, 822.2281) -> (1565, 837.9541)
  arc A200 (1567.1661, 839.9472) -> (1565, 837.9541) centre (1567, 837.9541) ccw
  line L282 (1567.1661, 839.9472) -> (1683.1661, 830.2805)
  arc A201 (1685, 828.2874) -> (1683.1661, 830.2805) centre (1683, 828.2874) ccw
  line L283 (1685, 828.2874) -> (1685, 822.2277)
  arc A202 (1683, 820.2277) -> (1685, 822.2277) centre (1683, 822.2277) ccw
  line L284 (1683, 820.2277) -> (1567, 820.2277)
  arc A203 (1565, 822.2281) -> (1567, 820.2277) centre (1567, 822.2277) ccw
  line L285 (1845, 1062.2281) -> (1845, 1077.9541)
  arc A204 (1847.1661, 1079.9472) -> (1845, 1077.9541) centre (1847, 1077.9541) ccw
  line L286 (1847.1661, 1079.9472) -> (1963.1661, 1070.2805)
  arc A205 (1965, 1068.2874) -> (1963.1661, 1070.2805) centre (1963, 1068.2874) ccw
  line L287 (1965, 1068.2874) -> (1965, 1062.2277)
  arc A206 (1963, 1060.2277) -> (1965, 1062.2277) centre (1963, 1062.2277) ccw
  line L288 (1963, 1060.2277) -> (1847, 1060.2277)
  arc A207 (1845, 1062.2281) -> (1847, 1060.2277) centre (1847, 1062.2277) ccw
  line L289 (1565, 742.2281) -> (1565, 757.9541)
  arc A208 (1567.1661, 759.9472) -> (1565, 757.9541) centre (1567, 757.9541) ccw
  line L290 (1567.1661, 759.9472) -> (1683.1661, 750.2805)
  arc A209 (1685, 748.2874) -> (1683.1661, 750.2805) centre (1683, 748.2874) ccw
  line L291 (1685, 748.2874) -> (1685, 742.2277)
  arc A210 (1683, 740.2277) -> (1685, 742.2277) centre (1683, 742.2277) ccw
  line L292 (1683, 740.2277) -> (1567, 740.2277)
  arc A211 (1565, 742.2281) -> (1567, 740.2277) centre (1567, 742.2277) ccw
  line L293 (1825.3322, 1112.9996) -> (1825.3322, 1097.2736)
  arc A212 (1823.1661, 1095.2805) -> (1825.3322, 1097.2736) centre (1823.3322, 1097.2736) ccw
  line L294 (1823.1661, 1095.2805) -> (1707.1661, 1104.9472)
  arc A213 (1705.3322, 1106.9403) -> (1707.1661, 1104.9472) centre (1707.3322, 1106.9403) ccw
  line L295 (1705.3322, 1106.9403) -> (1705.3322, 1113)
  arc A214 (1707.3322, 1115) -> (1705.3322, 1113) centre (1707.3322, 1113) ccw
  line L296 (1707.3322, 1115) -> (1823.3322, 1115)
  arc A215 (1825.3322, 1112.9996) -> (1823.3322, 1115) centre (1823.3322, 1113) ccw
  line L297 (1825.3322, 792.9996) -> (1825.3322, 777.2736)
  arc A216 (1823.1661, 775.2805) -> (1825.3322, 777.2736) centre (1823.3322, 777.2736) ccw
  line L298 (1823.1661, 775.2805) -> (1707.1661, 784.9472)
  arc A217 (1705.3322, 786.9403) -> (1707.1661, 784.9472) centre (1707.3322, 786.9403) ccw
  line L299 (1705.3322, 786.9403) -> (1705.3322, 793)
  arc A218 (1707.3322, 795) -> (1705.3322, 793) centre (1707.3322, 793) ccw
  line L300 (1707.3322, 795) -> (1823.3322, 795)
  arc A219 (1825.3322, 792.9996) -> (1823.3322, 795) centre (1823.3322, 793) ccw
  line L301 (1965.3322, 1112.9996) -> (1965.3322, 1097.2736)
  arc A220 (1963.1661, 1095.2805) -> (1965.3322, 1097.2736) centre (1963.3322, 1097.2736) ccw
  line L302 (1963.1661, 1095.2805) -> (1847.1661, 1104.9472)
  arc A221 (1845.3322, 1106.9403) -> (1847.1661, 1104.9472) centre (1847.3322, 1106.9403) ccw
  line L303 (1845.3322, 1106.9403) -> (1845.3322, 1113)
  arc A222 (1847.3322, 1115) -> (1845.3322, 1113) centre (1847.3322, 1113) ccw
  line L304 (1847.3322, 1115) -> (1963.3322, 1115)
  arc A223 (1965.3322, 1112.9996) -> (1963.3322, 1115) centre (1963.3322, 1113) ccw
  line L305 (1965.3322, 952.9996) -> (1965.3322, 937.2736)
  arc A224 (1963.1661, 935.2805) -> (1965.3322, 937.2736) centre (1963.3322, 937.2736) ccw
  line L306 (1963.1661, 935.2805) -> (1847.1661, 944.9472)
  arc A225 (1845.3322, 946.9403) -> (1847.1661, 944.9472) centre (1847.3322, 946.9403) ccw
  line L307 (1845.3322, 946.9403) -> (1845.3322, 953)
  arc A226 (1847.3322, 955) -> (1845.3322, 953) centre (1847.3322, 953) ccw
  line L308 (1847.3322, 955) -> (1963.3322, 955)
  arc A227 (1965.3322, 952.9996) -> (1963.3322, 955) centre (1963.3322, 953) ccw
  line L309 (1705, 822.2281) -> (1705, 837.9541)
  arc A228 (1707.1661, 839.9472) -> (1705, 837.9541) centre (1707, 837.9541) ccw
  line L310 (1707.1661, 839.9472) -> (1823.1661, 830.2805)
  arc A229 (1825, 828.2874) -> (1823.1661, 830.2805) centre (1823, 828.2874) ccw
  line L311 (1825, 828.2874) -> (1825, 822.2277)
  arc A230 (1823, 820.2277) -> (1825, 822.2277) centre (1823, 822.2277) ccw
  line L312 (1823, 820.2277) -> (1707, 820.2277)
  arc A231 (1705, 822.2281) -> (1707, 820.2277) centre (1707, 822.2277) ccw
  line L313 (1825.3322, 872.9996) -> (1825.3322, 857.2736)
  arc A232 (1823.1661, 855.2805) -> (1825.3322, 857.2736) centre (1823.3322, 857.2736) ccw
  line L314 (1823.1661, 855.2805) -> (1707.1661, 864.9472)
  arc A233 (1705.3322, 866.9403) -> (1707.1661, 864.9472) centre (1707.3322, 866.9403) ccw
  line L315 (1705.3322, 866.9403) -> (1705.3322, 873)
  arc A234 (1707.3322, 875) -> (1705.3322, 873) centre (1707.3322, 873) ccw
  line L316 (1707.3322, 875) -> (1823.3322, 875)
  arc A235 (1825.3322, 872.9996) -> (1823.3322, 875) centre (1823.3322, 873) ccw
  line L317 (1705, 742.2281) -> (1705, 757.9541)
  arc A236 (1707.1661, 759.9472) -> (1705, 757.9541) centre (1707, 757.9541) ccw
  line L318 (1707.1661, 759.9472) -> (1823.1661, 750.2805)
  arc A237 (1825, 748.2874) -> (1823.1661, 750.2805) centre (1823, 748.2874) ccw
  line L319 (1825, 748.2874) -> (1825, 742.2277)
  arc A238 (1823, 740.2277) -> (1825, 742.2277) centre (1823, 742.2277) ccw
  line L320 (1823, 740.2277) -> (1707, 740.2277)
  arc A239 (1705, 742.2281) -> (1707, 740.2277) centre (1707, 742.2277) ccw
  line L321 (1845, 917.9541) -> (1845, 902.2281)
  arc A240 (1845, 902.2281) -> (1847, 900.2277) centre (1847, 902.2277) ccw
  line L322 (1847, 900.2277) -> (1963, 900.2277)
  arc A241 (1963, 900.2277) -> (1965, 902.2277) centre (1963, 902.2277) ccw
  line L323 (1965, 902.2277) -> (1965, 908.2874)
  arc A242 (1965, 908.2874) -> (1963.1661, 910.2805) centre (1963, 908.2874) ccw
  line L324 (1963.1661, 910.2805) -> (1847.1661, 919.9472)
  arc A243 (1847.1661, 919.9472) -> (1845, 917.9541) centre (1847, 917.9541) ccw
  line L325 (1845, 757.9541) -> (1845, 742.2281)
  arc A244 (1845, 742.2281) -> (1847, 740.2277) centre (1847, 742.2277) ccw
  line L326 (1847, 740.2277) -> (1963, 740.2277)
  arc A245 (1963, 740.2277) -> (1965, 742.2277) centre (1963, 742.2277) ccw
  line L327 (1965, 742.2277) -> (1965, 748.2874)
  arc A246 (1965, 748.2874) -> (1963.1661, 750.2805) centre (1963, 748.2874) ccw
  line L328 (1963.1661, 750.2805) -> (1847.1661, 759.9472)
  arc A247 (1847.1661, 759.9472) -> (1845, 757.9541) centre (1847, 757.9541) ccw
  line L329 (1845, 982.2281) -> (1845, 997.9541)
  arc A248 (1847.1661, 999.9472) -> (1845, 997.9541) centre (1847, 997.9541) ccw
  line L330 (1847.1661, 999.9472) -> (1963.1661, 990.2805)
  arc A249 (1965, 988.2874) -> (1963.1661, 990.2805) centre (1963, 988.2874) ccw
  line L331 (1965, 988.2874) -> (1965, 982.2277)
  arc A250 (1963, 980.2277) -> (1965, 982.2277) centre (1963, 982.2277) ccw
  line L332 (1963, 980.2277) -> (1847, 980.2277)
  arc A251 (1845, 982.2281) -> (1847, 980.2277) centre (1847, 982.2277) ccw
  line L333 (1965.3322, 1032.9996) -> (1965.3322, 1017.2736)
  arc A252 (1963.1661, 1015.2805) -> (1965.3322, 1017.2736) centre (1963.3322, 1017.2736) ccw
  line L334 (1963.1661, 1015.2805) -> (1847.1661, 1024.9472)
  arc A253 (1845.3322, 1026.9403) -> (1847.1661, 1024.9472) centre (1847.3322, 1026.9403) ccw
  line L335 (1845.3322, 1026.9403) -> (1845.3322, 1033)
  arc A254 (1847.3322, 1035) -> (1845.3322, 1033) centre (1847.3322, 1033) ccw
  line L336 (1847.3322, 1035) -> (1963.3322, 1035)
  arc A255 (1965.3322, 1032.9996) -> (1963.3322, 1035) centre (1963.3322, 1033) ccw
  line L337 (1845, 837.9541) -> (1845, 822.2281)
  arc A256 (1845, 822.2281) -> (1847, 820.2277) centre (1847, 822.2277) ccw
  line L338 (1847, 820.2277) -> (1963, 820.2277)
  arc A257 (1963, 820.2277) -> (1965, 822.2277) centre (1963, 822.2277) ccw
  line L339 (1965, 822.2277) -> (1965, 828.2874)
  arc A258 (1965, 828.2874) -> (1963.1661, 830.2805) centre (1963, 828.2874) ccw
  line L340 (1963.1661, 830.2805) -> (1847.1661, 839.9472)
  arc A259 (1847.1661, 839.9472) -> (1845, 837.9541) centre (1847, 837.9541) ccw
  line L341 (1985, 742.2281) -> (1985, 757.9541)
  arc A260 (1987.1661, 759.9472) -> (1985, 757.9541) centre (1987, 757.9541) ccw
  line L342 (1987.1661, 759.9472) -> (2103.1661, 750.2805)
  arc A261 (2105, 748.2874) -> (2103.1661, 750.2805) centre (2103, 748.2874) ccw
  arc A262 (2103, 740.2277) -> (2105, 742.2277) centre (2103, 742.2277) ccw
  line L343 (2103, 740.2277) -> (1987, 740.2277)
  arc A263 (1985, 742.2281) -> (1987, 740.2277) centre (1987, 742.2277) ccw
  line L344 (2105.3322, 792.9996) -> (2105.3322, 777.2736)
  arc A264 (2103.1661, 775.2805) -> (2105.3322, 777.2736) centre (2103.3322, 777.2736) ccw
  line L345 (2103.1661, 775.2805) -> (1987.1661, 784.9472)
  arc A265 (1985.3322, 786.9403) -> (1987.1661, 784.9472) centre (1987.3322, 786.9403) ccw
  line L346 (1985.3322, 786.9403) -> (1985.3322, 793)
  arc A266 (1987.3322, 795) -> (1985.3322, 793) centre (1987.3322, 793) ccw
  line L347 (1987.3322, 795) -> (2103.3322, 795)
  arc A267 (2105.3322, 792.9996) -> (2103.3322, 795) centre (2103.3322, 793) ccw
  line L348 (2245.3322, 792.9996) -> (2245.3322, 777.2736)
  arc A268 (2243.1661, 775.2805) -> (2245.3322, 777.2736) centre (2243.3322, 777.2736) ccw
  line L349 (2243.1661, 775.2805) -> (2127.1661, 784.9472)
  arc A269 (2125.3322, 786.9403) -> (2127.1661, 784.9472) centre (2127.3322, 786.9403) ccw
  line L350 (2125.3322, 786.9403) -> (2125.3322, 793)
  arc A270 (2127.3322, 795) -> (2125.3322, 793) centre (2127.3322, 793) ccw
  line L351 (2127.3322, 795) -> (2243.3322, 795)
  arc A271 (2245.3322, 792.9996) -> (2243.3322, 795) centre (2243.3322, 793) ccw
  line L352 (2125, 757.9541) -> (2125, 742.2281)
  arc A272 (2125, 742.2281) -> (2127, 740.2277) centre (2127, 742.2277) ccw
  line L353 (2127, 740.2277) -> (2243, 740.2277)
  arc A273 (2243, 740.2277) -> (2245, 742.2277) centre (2243, 742.2277) ccw
  line L354 (2245, 742.2277) -> (2245, 748.2874)
  arc A274 (2245, 748.2874) -> (2243.1661, 750.2805) centre (2243, 748.2874) ccw
  line L355 (2243.1661, 750.2805) -> (2127.1661, 759.9472)
  arc A275 (2127.1661, 759.9472) -> (2125, 757.9541) centre (2127, 757.9541) ccw
  line L356 (2125, 837.9541) -> (2125, 822.2281)
  arc A276 (2125, 822.2281) -> (2127, 820.2277) centre (2127, 822.2277) ccw
  line L357 (2127, 820.2277) -> (2243, 820.2277)
  arc A277 (2243, 820.2277) -> (2245, 822.2277) centre (2243, 822.2277) ccw
  line L358 (2245, 822.2277) -> (2245, 828.2874)
  arc A278 (2245, 828.2874) -> (2243.1661, 830.2805) centre (2243, 828.2874) ccw
  line L359 (2243.1661, 830.2805) -> (2127.1661, 839.9472)
  arc A279 (2127.1661, 839.9472) -> (2125, 837.9541) centre (2127, 837.9541) ccw
  line L360 (1985, 902.2281) -> (1985, 917.9541)
  arc A280 (1987.1661, 919.9472) -> (1985, 917.9541) centre (1987, 917.9541) ccw
  line L361 (1987.1661, 919.9472) -> (2103.1661, 910.2805)
  arc A281 (2105, 908.2874) -> (2103.1661, 910.2805) centre (2103, 908.2874) ccw
  line L362 (2105, 908.2874) -> (2105, 902.2277)
  arc A282 (2103, 900.2277) -> (2105, 902.2277) centre (2103, 902.2277) ccw
  line L363 (2103, 900.2277) -> (1987, 900.2277)
  arc A283 (1985, 902.2281) -> (1987, 900.2277) centre (1987, 902.2277) ccw
  line L364 (2245.3322, 872.9996) -> (2245.3322, 857.2736)
  arc A284 (2243.1661, 855.2805) -> (2245.3322, 857.2736) centre (2243.3322, 857.2736) ccw
  line L365 (2243.1661, 855.2805) -> (2127.1661, 864.9472)
  arc A285 (2125.3322, 866.9403) -> (2127.1661, 864.9472) centre (2127.3322, 866.9403) ccw
  line L366 (2125.3322, 866.9403) -> (2125.3322, 873)
  arc A286 (2127.3322, 875) -> (2125.3322, 873) centre (2127.3322, 873) ccw
  line L367 (2127.3322, 875) -> (2243.3322, 875)
  arc A287 (2245.3322, 872.9996) -> (2243.3322, 875) centre (2243.3322, 873) ccw
  line L368 (2105.3322, 952.9996) -> (2105.3322, 937.2736)
  arc A288 (2103.1661, 935.2805) -> (2105.3322, 937.2736) centre (2103.3322, 937.2736) ccw
  line L369 (2103.1661, 935.2805) -> (1987.1661, 944.9472)
  arc A289 (1985.3322, 946.9403) -> (1987.1661, 944.9472) centre (1987.3322, 946.9403) ccw
  line L370 (1985.3322, 946.9403) -> (1985.3322, 953)
  arc A290 (1987.3322, 955) -> (1985.3322, 953) centre (1987.3322, 953) ccw
  line L371 (1987.3322, 955) -> (2103.3322, 955)
  arc A291 (2105.3322, 952.9996) -> (2103.3322, 955) centre (2103.3322, 953) ccw
  line L372 (2125, 902.2281) -> (2125, 917.9541)
  arc A292 (2127.1661, 919.9472) -> (2125, 917.9541) centre (2127, 917.9541) ccw
  line L373 (2127.1661, 919.9472) -> (2243.1661, 910.2805)
  arc A293 (2245, 908.2874) -> (2243.1661, 910.2805) centre (2243, 908.2874) ccw
  line L374 (2245, 908.2874) -> (2245, 902.2277)
  arc A294 (2243, 900.2277) -> (2245, 902.2277) centre (2243, 902.2277) ccw
  line L375 (2243, 900.2277) -> (2127, 900.2277)
  arc A295 (2125, 902.2281) -> (2127, 900.2277) centre (2127, 902.2277) ccw
  line L376 (2265, 997.9541) -> (2265, 982.2281)
  arc A296 (2265, 982.2281) -> (2267, 980.2277) centre (2267, 982.2277) ccw
  line L377 (2267, 980.2277) -> (2383, 980.2277)
  arc A297 (2383, 980.2277) -> (2385, 982.2277) centre (2383, 982.2277) ccw
  line L378 (2385, 982.2277) -> (2385, 988.2874)
  arc A298 (2385, 988.2874) -> (2383.1661, 990.2805) centre (2383, 988.2874) ccw
  line L379 (2383.1661, 990.2805) -> (2267.1661, 999.9472)
  arc A299 (2267.1661, 999.9472) -> (2265, 997.9541) centre (2267, 997.9541) ccw
  dimension "d1" = 30
  dimension "d3" = 179.25
  dimension "d5" = 149.25
  dimension "d7" = 358.5
  dimension "d9" = 1031.0789
  dimension "d11" = 450.1019
  dimension "d31" = 18
  dimension "d33" = 18
  dimension "d35" = 60
  constraints: 760 end point, 600 point on circle, 300 centre point
  measures "d1" distance between parallel lines of L126 L124
  measures "d3" distance from line of L122.end L124
  measures "d5" distance from line of L127.end L126
  measures "d7" distance of L116.end L117.end
  measures "d9" radius of A55
  measures "d11" radius of A56
  measures "d31" distance from line of L156.end L155
  measures "d33" distance from line of L124.end L123
  measures "d35" vertical distance of L129.end L127.end